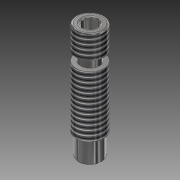
# Autodesk Inventor part: BREAK
Saved by Autodesk Inventor 2014 SP1 (Build 180222100, 222)
## iProperties
Created: 2017-07-08
Part Number: BREAK
Material: Типовые
Document SubType Name: Modeling
Designer: Stepan
Density: 1 g/cm^3
Appearance: Сталь — полированная
Author: Stepan
Autodesk Inventor part; units mm, degrees
ref_plane "YZ Plane" through (0, 0, 0) normal (1, 0, 0) x (0, 1, 0)
ref_plane "XZ Plane" through (0, 0, 0) normal (0, 1, 0) x (-1, 0, 0)
ref_plane "XY Plane" through (0, 0, 0) normal (0, 0, 1) x (1, 0, 0)
sketch "Эскиз1" plane through (0, 0, 0) normal (0, 1, 0) x (-1, 0, 0)
  line L0 (0, 0) -> (0, -25.3) construction
  line L1 (0, 0) -> (-3, 0) construction
  line L2 (-3, 0) -> (-3, -5)
  line L3 (0, -5) -> (-2.05, -5) construction
  line L4 (-2.05, -5) -> (-2.05, -7.1)
  line L5 (-3, -5) -> (-2.05, -5)
  line L6 (-2.05, -7.1) -> (-3, -7.1)
  line L7 (0, 0) -> (-1.6, 0) construction
  line L8 (-1.6, 0) -> (-3, 0) construction
  line L9 (-1.6, 0) -> (-3, 0)
  line L10 (-1.6, 0) -> (-1.6, -25.3)
  line L11 (0, -25.3) -> (-2.5, -25.3) construction
  line L12 (-1.6, -25.3) -> (-2.5, -25.3)
  line L13 (-2.5, -25.3) -> (-2.5, -20.3)
  line L14 (-2.5, -20.3) -> (-3, -20.3)
  line L15 (-3, -20.3) -> (-3, -7.1)
  dimension "d4" = 25.3
  dimension "d5" = 3
  dimension "d6" = 5
  dimension "d7" = 2.05
  dimension "d8" = 2.1
  dimension "d9" = 1.6
  dimension "d10" = 25.3
  dimension "d11" = 2.5
  dimension "d12" = 5
  constraints: 32 end point, 10 perpendicular, 2 parallel, 2 point on line, 1 collinear, 1 vertical
  measures "d4" distance of L0.start L0.end
  measures "d5" distance of L0.start L1.end
  measures "d6" distance of L1.end L2.end
  measures "d7" distance of L3.start L3.end
  measures "d8" distance of L3.end L4.end
  measures "d9" distance of L0.start L7.end
  measures "d10" distance of L7.end L10.end
  measures "d11" distance of L0.end L11.end
  measures "d12" distance of L11.end L13.end
revolve "Вращение1" add sketch "Эскиз1" angle 360 about axis through (0, 0, 0) along (0, 0, -1)
fillet "Сопряжение1" radius 0.4 4 edges at (-2.5, 0, -25.3) (-3, 0, 0) (-1.6, 0, 0) (-1.6, 0, -25.3)
thread "Резьба1" size "M6x1" class "6g" standard "ANSI Metric M Profile" full length
thread "Резьба2" size "M6x1" class "6g" standard "ANSI Metric M Profile" full length
